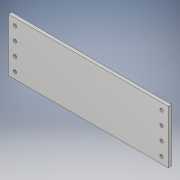
# Autodesk Inventor part: shortsides
Saved by Autodesk Inventor 2017 (Build 210142000, 142)
## iProperties
Created: 2017-07-28
Part Number: shortsides
Material: Generic
Document SubType Name: Modeling
Designer: Kai
Density: 1 g/cm^3
Appearance: Default
Author: Kai
Autodesk Inventor part; units mm, degrees
ref_plane "YZ Plane" through (0, 0, 0) normal (1, 0, 0) x (0, 1, 0)
ref_plane "XZ Plane" through (0, 0, 0) normal (0, 1, 0) x (-1, 0, 0)
ref_plane "XY Plane" through (0, 0, 0) normal (0, 0, 1) x (1, 0, 0)
sketch "Sketch1" plane through (0, 0, 0) normal (0, 0, 1) x (1, 0, 0)
  line L0 (0, 0) -> (-304.8, 0)
  line L1 (-304.8, 0) -> (-304.8, 101.6)
  line L2 (-304.8, 101.6) -> (0, 101.6)
  line L3 (0, 101.6) -> (0, 0)
  circle A0 centre (-292.1, 88.9) radius 3.1
  circle A1 centre (-292.1, 63.5) radius 3.1
  circle A2 centre (-292.1, 38.1) radius 3.1
  circle A3 centre (-292.1, 12.7) radius 3.1
  line L4 (-152.4, 101.6) -> (-152.4, 63.5) construction
  circle A4 centre (-12.7, 88.9) radius 3.1
  circle A5 centre (-12.7, 63.5) radius 3.1
  circle A6 centre (-12.7, 38.1) radius 3.1
  circle A7 centre (-12.7, 12.7) radius 3.1
  dimension "d0" = 304.8
  dimension "d1" = 101.6
  dimension "d2" = 6.2
  dimension "d3" = 12.7
  dimension "d4" = 12.7
  dimension "d7" = 25.4
  constraints: 10 end point, 8 centre point, 4 symmetric about line, 2 parallel, 2 vertical, 1 horizontal, 1 midpoint, 1 perpendicular, 10 other
  measures "d0" distance of L1.end L2.end
  measures "d1" distance of L0.end L1.end
  measures "d2" diameter of A0
  measures "d3" distance from line of A0.centre L1
  measures "d4" distance from line of L2 A0.centre
  measures "d7" distance of A0.centre A1.centre
extrude "Extrusion1" add sketch "Sketch1" along normal blind 6.35
body "Solid1"
